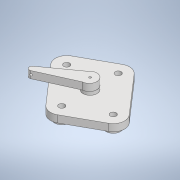
# Autodesk Inventor part: torque_calibrator
Saved by Autodesk Inventor 2021 (Build 250183000, 183)
## iProperties
Created: 2021-02-16
Part Number: torque_calibrator
Material: 일반
Document SubType Name: Modeling
Designer: jun85
Density: 1 g/cm^3
Appearance: 기본값
Author: jun85
Autodesk Inventor part; units mm, degrees
ref_plane "YZ Plane" through (0, 0, 0) normal (1, 0, 0) x (0, 1, 0)
ref_plane "XZ Plane" through (0, 0, 0) normal (0, 1, 0) x (-1, 0, 0)
ref_plane "XY Plane" through (0, 0, 0) normal (0, 0, 1) x (1, 0, 0)
sketch "스케치1" plane through (0, 0, 0) normal (0, 1, 0) x (-1, 0, 0)
  line L0 (23.5, 7) -> (-23.5, 7) construction
  line L1 (-23.5, 7) -> (-23.5, -7) construction
  line L2 (-23.5, -7) -> (23.5, -7) construction
  line L3 (23.5, -7) -> (23.5, 7) construction
  line L4 (23.5, 7) -> (-23.5, -7) construction
  line L5 (-23.5, 7) -> (23.5, -7) construction
  circle A0 centre (23.5, -7) radius 2.1
  circle A1 centre (0, -20) radius 2.1
  circle A2 centre (-23.5, 7) radius 2.1
  circle A3 centre (0, 20) radius 2.1
  line L6 (45.443, 0) -> (-45.443, 0) projected
  arc A4 (-6.0344, -25.2522) -> (3.8725, -27.0003) centre (0, -20) ccw
  arc A5 (-27.3725, 14.0003) -> (-29.5344, 1.7478) centre (-23.5, 7) ccw
  arc A6 (6.0344, 25.2522) -> (-3.8725, 27.0003) centre (0, 20) ccw
  line L7 (29.5344, -1.7478) -> (6.0344, 25.2522)
  line L8 (3.8725, -27.0003) -> (27.3725, -14.0003)
  line L9 (-3.8725, 27.0003) -> (-27.3725, 14.0003)
  line L10 (-29.5344, 1.7478) -> (-6.0344, -25.2522)
  arc A7 (27.3725, -14.0003) -> (29.5344, -1.7478) centre (23.5, -7) ccw
  point P0 (0, 0)
  point P1 (0, 0)
  point P2 (0, 0)
  point P3 (28.0132, 0)
  point P4 (-26.1926, 0)
  point P5 (-26.1926, 0)
  point P6 (-28.0132, 0)
  dimension "d0" = 4.2
  dimension "d1" = 47
  dimension "d2" = 14
  dimension "d3" = 40
  dimension "d7" = 8
  constraints: 20 end point, 8 centre point, 8 point on circle, 8 tangent, 6 coincident, 6 equal radius, 4 midpoint, 2 parallel, 2 vertical alignment, 1 horizontal, 1 perpendicular, 1 other
  measures "d0" diameter of A0
  measures "d1" distance of L1.end L2.end
  measures "d2" distance of L0.end L1.end
  measures "d3" distance of A3.centre A1.centre
  measures "d7" radius of A7
extrude "돌출1" add sketch "스케치1" along normal blind 5
sketch "스케치2" plane through (0, 0, 0) normal (0, -1, 0) x (1, 0, 0)
  circle A0 centre (-23.5, -7) radius 2.1 projected
  circle A1 centre (0, 20) radius 2.1 projected
  circle A2 centre (23.5, 7) radius 2.1 projected
  circle A3 centre (0, -20) radius 2.1 projected
  circle A4 centre (-23.5, -7) radius 5.1
  circle A5 centre (0, 20) radius 5.1
  circle A6 centre (23.5, 7) radius 5.1
  circle A7 centre (0, -20) radius 5.1
  point P0 (0, 0)
  dimension "d8" = 3
  constraints: 4 centre point, 4 coincident, 3 equal radius
  measures "d8" radial gap between concentric circles of A4 A0
extrude "돌출2" add sketch "스케치2" along normal blind 3
fillet "모깎기1" radius 3 4 edges at (-28.6, 0, -7) (-5.1, 0, -20) (-5.1, 0, 20) (18.4, 0, 7)
sketch "스케치3" plane through (0, 5, 0) normal (0, 1, 0) x (1, 0, 0)
  circle A0 centre (0, 0) radius 5
  dimension "d12" = 10
  constraints: 1 centre point, 1 coincident
  measures "d12" diameter of A0
extrude "돌출3" add sketch "스케치3" along normal blind 5
sketch "스케치4" plane through (0, 10, 0) normal (0, 1, 0) x (1, 0, 0)
  circle A0 centre (0, 0) radius 5 projected
  line L0 (0, 0) -> (25.9808, -15) construction
  line L1 (0, -5.4844) -> (25.159, -16.8234)
  line L2 (27.149, -13.3766) -> (4.7496, 2.7422)
  arc A1 (25.159, -16.8234) -> (27.149, -13.3766) centre (25.9808, -15) ccw
  line L3 (0, 0) -> (0, 30) construction
  line L4 (4.7496, 2.7422) -> (1.99, 30.2)
  line L5 (-1.99, 30.2) -> (-4.7496, 2.7422)
  arc A2 (1.99, 30.2) -> (-1.99, 30.2) centre (0, 30) ccw
  line L6 (0, 0) -> (-25.9808, -15) construction
  line L7 (-4.7496, 2.7422) -> (-27.149, -13.3766)
  line L8 (-25.159, -16.8234) -> (0, -5.4844)
  arc A3 (-27.149, -13.3766) -> (-25.159, -16.8234) centre (-25.9808, -15) ccw
  circle A4 centre (0, 0) radius 5 projected
  line L9 (25.9808, -15) -> (-25.9808, -15) construction
  line L10 (-25.9808, -15) -> (0, 30) construction
  line L11 (0, 30) -> (25.9808, -15) construction
  line L12 (4.7496, 2.7422) -> (0, -5.4844) construction
  line L13 (0, -5.4844) -> (-4.7496, 2.7422) construction
  line L14 (-4.7496, 2.7422) -> (4.7496, 2.7422) construction
  line L15 (5, 30.75) -> (-5, 30.75)
  line L16 (-5, 30.75) -> (-5, 29.25)
  line L17 (-5, 29.25) -> (5, 29.25)
  line L18 (5, 29.25) -> (5, 30.75)
  line L19 (5, 30.75) -> (-5, 29.25) construction
  line L20 (-5, 30.75) -> (5, 29.25) construction
  line L21 (-29.1303, -11.0449) -> (-24.1303, -19.7051)
  line L22 (-24.1303, -19.7051) -> (-22.8312, -18.9551)
  line L23 (-22.8312, -18.9551) -> (-27.8312, -10.2949)
  line L24 (-27.8312, -10.2949) -> (-29.1303, -11.0449)
  line L25 (-29.1303, -11.0449) -> (-22.8312, -18.9551) construction
  line L26 (-24.1303, -19.7051) -> (-27.8312, -10.2949) construction
  line L27 (27.8312, -10.2949) -> (22.8312, -18.9551)
  line L28 (22.8312, -18.9551) -> (24.1303, -19.7051)
  line L29 (24.1303, -19.7051) -> (29.1303, -11.0449)
  line L30 (29.1303, -11.0449) -> (27.8312, -10.2949)
  line L31 (27.8312, -10.2949) -> (24.1303, -19.7051) construction
  line L32 (22.8312, -18.9551) -> (29.1303, -11.0449) construction
  line L33 (0, 44) -> (0, -40) projected
  circle A5 centre (0, 20) radius 2.1 projected
  circle A6 centre (0, 20) radius 6.5
  circle A7 centre (0, 20) radius 4
  arc A8 (0, -5.4844) -> (-4.7496, 2.7422) centre (-0.284, -0.164) ccw
  point P0 (12.9904, -7.5)
  point P1 (0, 15)
  point P2 (-12.9904, -7.5)
  point P3 (0, 30)
  point P4 (0, 30)
  point P5 (3.5616, 14.5626)
  point P6 (2.4083, 26.0374)
  point P7 (3.7599, 25.3021)
  point P8 (-0.4655, 13.5167)
  dimension "d15" = 30
  dimension "d17" = 2
  dimension "d18" = 10
  dimension "d19" = 1.5
  dimension "d29" = 13
  dimension "d30" = 8
  constraints: 72 end point, 10 midpoint, 8 point on circle, 8 tangent, 7 parallel, 6 centre point, 6 perpendicular, 4 coincident, 4 equal length, 2 equal radius, 2 point on line, 1 horizontal, 14 other
  measures "d15" distance of L0.start L0.end
  measures "d17" radius of A2
  measures "d18" distance of L16.end L17.end
  measures "d19" distance of L17.end L15.start
  measures "d29" diameter of A6
  measures "d30" diameter of A7
extrude "돌출4" add sketch "스케치4" along normal mid plane 5 contours A0 L33 | A0 A8 L33 | A0 L33 A8 | L33 L8 L23 L7 A8 A0 | A0 L33 | L8 A3 L21 L7 L23 | A3 L21
extrude "돌출5" cut sketch "스케치4" along normal mid plane 1.5 contours L27 L2 A1 L29 L1 | L1 A1 L29 L28 L27 | L23 L22 L21 A3 L8 | L8 A3 L21 L7 L23 | L27 L30 L29 A1 L2 | L7 A3 L21 L24 L23 | L17 L16 L15 A2 L5 | L5 A2 L15 L33 L17 | L33 L15 A2 L4 L17 | L4 A2 L15 L18 L17
fillet "모깎기2" radius 0.75 4 edges at (-25.3312, 9.25, 14.625) (-25.3312, 10.75, 14.625) (-26.6303, 9.25, 15.375) (-26.6303, 10.75, 15.375)
sketch "스케치5" plane through (0, 12.5, 0) normal (0, 1, 0) x (1, 0, 0)
  circle A0 centre (0, 0) radius 0.75
  dimension "d25" = 1.5
  constraints: 1 centre point, 1 coincident
  measures "d25" diameter of A0
extrude "돌출6" cut sketch "스케치5" against normal through all
